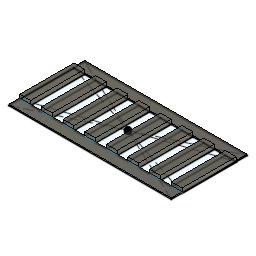
50mm Filter Grate Top (Autodesk Fusion 360 design; units mm, degrees)
Autodesk Fusion 360 part; units mm, degrees
note: some values were not read from the file. Chosen so that the rebuilt part matches the saved one: which bodies a step acts on.
sketch "Sketch1" plane through (0, 0, 0) normal (0, 0, 1) x (1, 0, 0)
  line L0 (75, -35) -> (-75, -35)
  line L1 (-75, -35) -> (-75, 35)
  line L2 (-75, 35) -> (75, 35)
  line L3 (75, 35) -> (75, -35)
  line L4 (75, -35) -> (-75, 35) construction
  line L5 (-75, -35) -> (75, 35) construction
  line L6 (75, -25) -> (-75, -25)
  line L7 (-75, -25) -> (-75, 25)
  line L8 (-75, 25) -> (75, 25)
  line L9 (75, 25) -> (75, -25)
  line L10 (75, -25) -> (-75, 25) construction
  line L11 (-75, -25) -> (75, 25) construction
  line L12 (-75, 25) -> (-65, 25)
  line L13 (-65, 25) -> (-65, -25)
  line L14 (-65, -25) -> (-75, -25)
  line L15 (-75, -25) -> (-75, 25)
  line L16 (-55, 25) -> (-45, 25)
  line L17 (-45, 25) -> (-45, -25)
  line L18 (-45, -25) -> (-55, -25)
  line L19 (-55, -25) -> (-55, 25)
  line L20 (-35, 25) -> (-25, 25)
  line L21 (-25, 25) -> (-25, -25)
  line L22 (-25, -25) -> (-35, -25)
  line L23 (-35, -25) -> (-35, 25)
  line L24 (-15, 25) -> (-5, 25)
  line L25 (-5, 25) -> (-5, -25)
  line L26 (-5, -25) -> (-15, -25)
  line L27 (-15, -25) -> (-15, 25)
  line L28 (5, 25) -> (15, 25)
  line L29 (15, 25) -> (15, -25)
  line L30 (15, -25) -> (5, -25)
  line L31 (5, -25) -> (5, 25)
  line L32 (25, 25) -> (35, 25)
  line L33 (35, 25) -> (35, -25)
  line L34 (35, -25) -> (25, -25)
  line L35 (25, -25) -> (25, 25)
  line L36 (45, 25) -> (55, 25)
  line L37 (55, 25) -> (55, -25)
  line L38 (55, -25) -> (45, -25)
  line L39 (45, -25) -> (45, 25)
  line L40 (65, 25) -> (75, 25)
  line L41 (75, 25) -> (75, -25)
  line L42 (75, -25) -> (65, -25)
  line L43 (65, -25) -> (65, 25)
  dimension "d1" = 150
  dimension "d2" = 70
  dimension "d3" = 150
  dimension "d4" = 50
  dimension "d5" = 10
  dimension "d8" = 140
  dimension "d9" = 0
  constraint horizontal L0
  constraint perpendicular L0 L1
  constraint parallel L0 L2
  constraint parallel L1 L3
  constraint coincident L4 origin
  constraint coincident L5 origin
  constraint horizontal L6
  constraint perpendicular L6 L7
  constraint parallel L6 L8
  constraint parallel L7 L9
  constraint coincident L10 origin
  constraint coincident L11 origin
  constraint horizontal L12
  constraint vertical L13
  constraint horizontal L14
  constraint vertical L15
  measures "d1" distance of L1.end L2.end
  measures "d2" distance of L0.end L1.end
  measures "d3" distance of L7.end L8.end
  measures "d4" distance of L6.end L7.end
  measures "d5" distance of L7.end L12.end
extrude "Extrude1" add sketch "Sketch1" along normal blind 4 contours L3 L6 L8 L9 L40 L41 L42 L43 | L1 L6 L7 L8 L12 L13 L14 L15 | L6 L8 L36 L37 L38 L39 | L6 L8 L16 L17 L18 L19 | L6 L8 L32 L33 L34 L35 | L6 L8 L20 L21 L22 L23 | L6 L8 L28 L29 L30 L31 | L6 L8 L24 L25 L26 L27 makes body 1 at (51.6667, -8.3333, 0) makes body 2 at (-71.6667, 8.3333, 0) makes body 3 at (31.6667, -8.3333, 0) makes body 4 at (-51.6667, 8.3333, 0) makes body 5 at (68.3333, -8.3333, 0) makes body 6 at (-31.6667, 8.3333, 0) makes body 7 at (11.6667, -8.3333, 0) makes body 8 at (-11.6667, 8.3333, 0)
extrude "Extrude2" add sketch "Sketch1" along normal blind 1 contours L0 L1 L3 L6 L14 L18 L22 L26 L30 L34 L38 L42 | L1 L2 L3 L8 L12 L16 L20 L24 L28 L32 L36 L40 bodies 1 2 3 4 5 6 7 8
